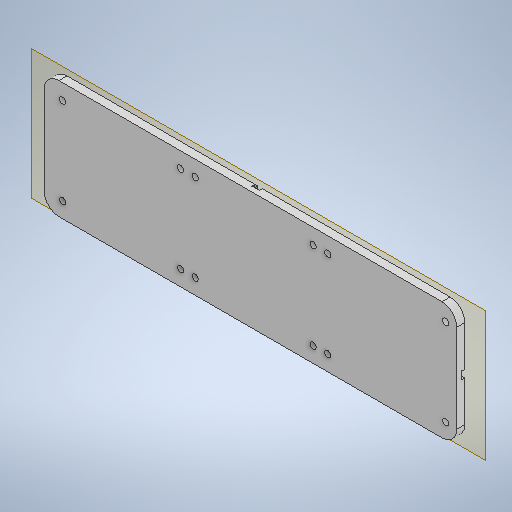
# Autodesk Inventor part: led 7 seg with sec v3 bottom
Saved by Autodesk Inventor 2026 (Build 300175000, 175)
## iProperties
Created: 2025-08-14
Part Number: led 7 seg with sec v3 bottom
Material: Generic
Document SubType Name: Modeling
Designer: Korobeynikov
Density: 1 g/cm^3
Appearance: Default
Author: Korobeynikov
Autodesk Inventor part; units mm, degrees
ref_plane "YZ Plane" through (0, 0, 0) normal (1, 0, 0) x (0, 1, 0)
ref_plane "XZ Plane" through (0, 0, 0) normal (0, 1, 0) x (-1, 0, 0)
ref_plane "XY Plane" through (0, 0, 0) normal (0, 0, 1) x (1, 0, 0)
ref_plane "Work Plane1" through (0, 0, 0) normal (0, 0, 1) x (1, 0, 0)
sketch "Sketch1" plane through (0, 0, 0) normal (0, 0, 1) x (1, 0, 0)
  line L0 (-130, -40) -> (130, -40) projected
  arc A0 (130, -40) -> (140, -30) centre (130, -30) ccw projected
  line L1 (140, -30) -> (140, 30) projected
  arc A1 (140, 30) -> (130, 40) centre (130, 30) ccw projected
  line L2 (130, 40) -> (-130, 40) projected
  arc A2 (-130, 40) -> (-140, 30) centre (-130, 30) ccw projected
  line L3 (-140, 30) -> (-140, -30) projected
  arc A3 (-140, -30) -> (-130, -40) centre (-130, -30) ccw projected
  arc A4 (130, -38) -> (138, -30) centre (130, -30) ccw projected
  line L4 (130, -38) -> (-130, -38) projected
  arc A5 (-138, -30) -> (-130, -38) centre (-130, -30) ccw projected
  line L5 (-138, -30) -> (-138, 30) projected
  arc A6 (-130, 38) -> (-138, 30) centre (-130, 30) ccw projected
  line L6 (-130, 38) -> (130, 38) projected
  arc A7 (138, 30) -> (130, 38) centre (130, 30) ccw projected
  line L7 (138, 30) -> (138, -30) projected
  circle A8 centre (132.5, 29.5) radius 2.15 projected
  circle A9 centre (132.5, -29.5) radius 2.15 projected
  circle A10 centre (52.5, 29.5) radius 2.15 projected
  circle A11 centre (42.5, 29.5) radius 2.15 projected
  circle A12 centre (42.5, -29.5) radius 2.15 projected
  circle A13 centre (52.5, -29.5) radius 2.15 projected
  circle A14 centre (-37.5, 29.5) radius 2.15 projected
  circle A15 centre (-37.5, -29.5) radius 2.15 projected
  circle A16 centre (-47.5, -29.5) radius 2.15 projected
  circle A17 centre (-47.5, 29.5) radius 2.15 projected
  circle A18 centre (-127.5, 29.5) radius 2.15 projected
  circle A19 centre (-127.5, -29.5) radius 2.15 projected
  point P0 (0, 0)
extrude "Extrusion1" add sketch "Sketch1" along normal blind 4 contours A3 L3 A2 L2 A1 L1 A0 L0
sketch "Sketch2" plane through (0, 0, 4) normal (0, 0, 1) x (1, 0, 0)
  arc A0 (130, -40) -> (140, -30) centre (130, -30) ccw projected
  line L0 (140, -30) -> (140, 30) projected
  arc A1 (140, 30) -> (130, 40) centre (130, 30) ccw projected
  line L1 (130, 40) -> (-130, 40) projected
  arc A2 (-130, 40) -> (-140, 30) centre (-130, 30) ccw projected
  line L2 (-140, 30) -> (-140, -30) projected
  arc A3 (-140, -30) -> (-130, -40) centre (-130, -30) ccw projected
  line L3 (-130, -40) -> (130, -40) projected
  line L4 (-138, -30) -> (-138, 30) projected
  arc A4 (-130, 38) -> (-138, 30) centre (-130, 30) ccw projected
  line L5 (-130, 38) -> (130, 38) projected
  arc A5 (138, 30) -> (130, 38) centre (130, 30) ccw projected
  line L6 (138, 30) -> (138, -30) projected
  arc A6 (130, -38) -> (138, -30) centre (130, -30) ccw projected
  line L7 (130, -38) -> (-130, -38) projected
  arc A7 (-138, -30) -> (-130, -38) centre (-130, -30) ccw projected
  circle A8 centre (-127.5, 29.5) radius 2.15 projected
  circle A9 centre (-127.5, -29.5) radius 2.15 projected
  circle A10 centre (-47.5, -29.5) radius 2.15 projected
  circle A11 centre (-47.5, 29.5) radius 2.15 projected
  circle A12 centre (-37.5, 29.5) radius 2.15 projected
  circle A13 centre (-37.5, -29.5) radius 2.15 projected
  circle A14 centre (42.5, -29.5) radius 2.15 projected
  circle A15 centre (42.5, 29.5) radius 2.15 projected
  circle A16 centre (52.5, 29.5) radius 2.15 projected
  circle A17 centre (52.5, -29.5) radius 2.15 projected
  circle A18 centre (132.5, 29.5) radius 2.15 projected
  circle A19 centre (132.5, -29.5) radius 2.15 projected
  point P0 (0, 0)
extrude "Extrusion2" add sketch "Sketch2" along normal blind 1.5 contours L3 A3 L2 A2 L1 A1 L0 A0 | L4 A4 L5 A5 L6 A6 L7 A7
sketch "Sketch3" plane through (0, 0, 4) normal (0, 0, -1) x (-1, 0, 0)
  circle A0 centre (-132.5, 29.5) radius 2.15 projected
  circle A1 centre (-132.5, 29.5) radius 4.5
  circle A2 centre (-132.5, -29.5) radius 2.15 projected
  circle A3 centre (-132.5, -29.5) radius 4.5
  circle A4 centre (-52.5, 29.5) radius 2.15 projected
  circle A5 centre (-52.5, 29.5) radius 4.5
  circle A6 centre (-42.5, 29.5) radius 2.15 projected
  circle A7 centre (-42.5, 29.5) radius 4.5
  circle A8 centre (-52.5, -29.5) radius 2.15 projected
  circle A9 centre (-52.5, -29.5) radius 4.5
  circle A10 centre (-42.5, -29.5) radius 2.15 projected
  circle A11 centre (-42.5, -29.5) radius 4.5
  circle A12 centre (37.5, 29.5) radius 2.15 projected
  circle A13 centre (37.5, 29.5) radius 4.5
  circle A14 centre (47.5, 29.5) radius 2.15 projected
  circle A15 centre (47.5, 29.5) radius 4.5
  circle A16 centre (37.5, -29.5) radius 2.15 projected
  circle A17 centre (37.5, -29.5) radius 4.5
  circle A18 centre (47.5, -29.5) radius 2.15 projected
  circle A19 centre (47.5, -29.5) radius 4.5
  circle A20 centre (127.5, -29.5) radius 2.15 projected
  circle A21 centre (127.5, -29.5) radius 4.5
  circle A22 centre (127.5, 29.5) radius 2.15 projected
  circle A23 centre (127.5, 29.5) radius 4.5
  point P0 (0, 0)
  dimension "d4" = 9
  constraints: 12 centre point, 12 coincident, 11 equal radius
  measures "d4" diameter of A1
extrude "Extrusion3" add sketch "Sketch3" along normal blind 2
sketch "Sketch4" plane through (0, 0, 4) normal (0, 0, -1) x (-1, 0, 0)
  line L0 (-116.4072, -36) -> (-66.4072, -36)
  line L1 (-66.4072, -36) -> (-66.4072, -38)
  line L2 (-66.4072, -38) -> (-116.4072, -38)
  line L3 (-116.4072, -38) -> (-116.4072, -36)
  circle A0 centre (-132.5, -29.5) radius 2.15 projected
  line L4 (-132.5, -29.5) -> (-50.3144, -29.5)
  line L5 (-130, -38) -> (130, -38) projected
  line L6 (0, 0) -> (-95.519, 0)
  line L7 (-116.4072, 36) -> (-66.4072, 36)
  line L8 (-66.4072, 36) -> (-66.4072, 38)
  line L9 (-66.4072, 38) -> (-116.4072, 38)
  line L10 (-116.4072, 38) -> (-116.4072, 36)
  line L11 (-26.4072, 36) -> (23.5928, 36)
  line L12 (23.5928, 36) -> (23.5928, 38)
  line L13 (23.5928, 38) -> (-26.4072, 38)
  line L14 (-26.4072, 38) -> (-26.4072, 36)
  line L15 (-26.4072, -36) -> (23.5928, -36)
  line L16 (23.5928, -38) -> (-26.4072, -38)
  line L17 (-26.4072, -38) -> (-26.4072, -36)
  line L18 (23.5928, -36) -> (23.5928, -38)
  line L19 (63.5928, 36) -> (113.5928, 36)
  line L20 (113.5928, 36) -> (113.5928, 38)
  line L21 (113.5928, 38) -> (63.5928, 38)
  line L22 (63.5928, 38) -> (63.5928, 36)
  line L23 (63.5928, -36) -> (113.5928, -36)
  line L24 (113.5928, -38) -> (63.5928, -38)
  line L25 (63.5928, -38) -> (63.5928, -36)
  line L26 (113.5928, -36) -> (113.5928, -38)
  line L27 (136, 25) -> (138, 25)
  line L28 (138, 25) -> (138, -25)
  line L29 (138, -25) -> (136, -25)
  line L30 (136, -25) -> (136, 25)
  line L31 (138, -30) -> (138, 30) projected
  point P0 (-91.4072, -29.5)
  point P1 (-91.4072, -36)
  point P2 (-91.4072, -38)
  point P3 (-91.4072, 36)
  point P4 (-91.4072, 38)
  point P5 (-1.4072, 36)
  point P6 (-1.4072, 38)
  point P7 (-1.4072, -36)
  point P8 (-1.4072, -38)
  point P9 (88.5928, 36)
  point P10 (88.5928, 38)
  point P11 (88.5928, -36)
  point P12 (88.5928, -38)
  point P13 (138, 0)
  dimension "d7" = 2
  dimension "d8" = 50
  dimension "d11" = 90
  dimension "d18" = 72
  constraints: 60 end point, 6 symmetric about line, 5 horizontal, 5 midpoint, 4 parallel, 4 perpendicular, 1 point on line, 1 vertical alignment, 40 other
  measures "d7" distance of L2.end L0.start
  measures "d8" distance of L0.start L0.end
  measures "d11" distance of L7.start L11.start
  measures "d18" distance between parallel lines of L0 L7
extrude "Extrusion4" add sketch "Sketch4" along normal blind 6 contours L25 L23 L26 L5 | L17 L15 L18 L5 | L0 L1 L2 L3 | L10 L9 L8 L7 | L14 L13 L12 L11 | L22 L21 L20 L19 | L27 L28 L29 L30
sketch "Sketch5" plane through (0, 0, -2) normal (0, 0, -1) x (-1, 0, 0)
  line L0 (136, -2.5) -> (140, -2.5)
  line L1 (140, -2.5) -> (140, 2.5)
  line L2 (140, 2.5) -> (136, 2.5)
  line L3 (136, 2.5) -> (136, -2.5)
  line L4 (140, 30) -> (140, -30) projected
  line L5 (136, 25) -> (136, -25) projected
  line L6 (-2.5, 36) -> (2.5, 36)
  line L7 (2.5, 36) -> (2.5, 40)
  line L8 (2.5, 40) -> (-2.5, 40)
  line L9 (-2.5, 40) -> (-2.5, 36)
  line L10 (-2.5, -36) -> (2.5, -36)
  line L11 (2.5, -36) -> (2.5, -40)
  line L12 (2.5, -40) -> (-2.5, -40)
  line L13 (-2.5, -40) -> (-2.5, -36)
  line L14 (-140, 2.5) -> (-138, 2.5)
  line L15 (-138, 2.5) -> (-138, -2.5)
  line L16 (-138, -2.5) -> (-140, -2.5)
  line L17 (-140, -2.5) -> (-140, 2.5)
  line L18 (-130, 40) -> (130, 40) projected
  line L19 (130, -40) -> (-130, -40) projected
  line L20 (-140, -30) -> (-140, 30) projected
  line L21 (-138, 30) -> (-138, -30) projected
  line L22 (-26.4072, 36) -> (23.5928, 36) projected
  line L23 (23.5928, -36) -> (-26.4072, -36) projected
  point P0 (0, 0)
  point P1 (138, -2.5)
  point P2 (136, 0)
  point P3 (0, 40)
  point P4 (0, -40)
  point P5 (-140, 0)
  point P6 (-138, 0)
  point P7 (0, 36)
  point P8 (0, -36)
  dimension "d19" = 5
  constraints: 32 end point, 13 midpoint, 8 parallel, 4 horizontal, 4 perpendicular, 4 point on line, 3 equal length
  measures "d19" distance from line of L2 point (138, -2.5)
extrude "Extrusion5" cut sketch "Sketch5" against normal blind 4
body "Solid1"
